Autodesk Fusion 360 part; units mm, degrees
(part 3 of 5)
fillet "Fillet8" radius 2.5 2 edges at (-19.3, 26.725, 15) (19.3, 26.725, 15)
fillet "Fillet9" radius 2.5 4 edges at (20.0322, 25.9928, 10) (19.3, 24, 10) (-19.3, 24, 10) (-20.0322, 25.9928, 10)
fillet "Fillet10" radius 15 2 edges at (29.0855, 18.4895, 0) (-29.0855, 18.4895, 0)
sketch "Sketch20" plane through (0, 26.725, 0) normal (0, 1, 0) x (-1, 0, 0)
  line L0 (-21.8, 12.5) -> (-21.8, 20)
  line L1 (-21.8, 20) -> (-28.05, 20)
  line L2 (-28.05, 20) -> (-28.05, -20)
  line L3 (-28.05, -20) -> (28.05, -20)
  line L4 (28.05, -20) -> (28.05, 20)
  line L5 (28.05, 20) -> (21.8, 20)
  line L6 (21.8, 20) -> (21.8, 12.5)
  spline S0 degree 3 poles (17.4699, 10) (17.7885, 10) (18.1326, 10.0486) (18.7976, 10.2365) (19.1187, 10.3749) (19.8306, 10.7581) (20.2629, 11.0723) (21.0731, 11.7716) (21.4536, 12.1536) (21.8, 12.5) knots 1.263831 1.263831 1.263831 1.263831 1.35941 1.35941 1.454989 1.454989 1.601942 1.601942 1.748896 1.748896 1.748896 1.748896
  line L7 (17.4699, 10) -> (-17.4699, 10)
  spline S1 degree 3 poles (-21.8, 12.5) (-21.4536, 12.1536) (-21.0731, 11.7716) (-20.2629, 11.0723) (-19.8306, 10.7581) (-19.1187, 10.3749) (-18.7976, 10.2365) (-18.1326, 10.0486) (-17.7885, 10) (-17.4699, 10) knots 0 0 0 0 0.146954 0.146954 0.293907 0.293907 0.389486 0.389486 0.485065 0.485065 0.485065 0.485065
  line L8 (20, -20) -> (-20, -20)
  line L9 (-20, -20) -> (-20, -15)
  line L10 (-20, -15) -> (20, -15)
  line L11 (20, -15) -> (20, -20)
  dimension "d224" = 5
  dimension "d225" = 40
  dimension "d226" = 20
  constraint horizontal L8
  constraint vertical L9
  constraint horizontal L10
  constraint vertical L11
  constraint coincident L3 L8.start
  measures "d224" distance of L8 L10
  measures "d225" distance of L9 L11
  measures "d226" distance of origin L9
extrude "Extrude19" add sketch "Sketch20" along normal blind 7.05 contours L3 L8 L9 L10 L11
fillet "Fillet11" radius 2.5 2 edges at (-20, 26.725, -17.5) (-20, 33.775, -17.5)
fillet "Fillet11" radius 2.5 2 edges at (20, 33.775, -17.5) (20, 26.725, -17.5)
fillet "Fillet12" radius 2.5 1 edges at (0, 26.725, -15)
sketch "Sketch21" plane through (0, 26.725, 0) normal (0, 1, 0) x (-1, 0, 0)
  line L0 (22.5, -12.5) -> (22.5, -20)
  line L1 (22.5, -20) -> (28.05, -20)
  line L2 (28.05, -20) -> (28.05, 20)
  line L3 (28.05, 20) -> (21.8, 20)
  line L4 (21.8, 20) -> (21.8, 12.5)
  spline S0 degree 3 poles (17.4699, 10) (17.7885, 10) (18.1326, 10.0486) (18.7976, 10.2365) (19.1187, 10.3749) (19.8306, 10.7581) (20.2629, 11.0723) (21.0731, 11.7716) (21.4536, 12.1536) (21.8, 12.5) knots 1.263831 1.263831 1.263831 1.263831 1.35941 1.35941 1.454989 1.454989 1.601942 1.601942 1.748896 1.748896 1.748896 1.748896
  line L5 (17.4699, 10) -> (-17.4699, 10)
  spline S1 degree 3 poles (-21.8, 12.5) (-21.4536, 12.1536) (-21.0731, 11.7716) (-20.2629, 11.0723) (-19.8306, 10.7581) (-19.1187, 10.3749) (-18.7976, 10.2365) (-18.1326, 10.0486) (-17.7885, 10) (-17.4699, 10) knots 0 0 0 0 0.146954 0.146954 0.293907 0.293907 0.389486 0.389486 0.485065 0.485065 0.485065 0.485065
  line L6 (-21.8, 12.5) -> (-21.8, 20)
  line L7 (-21.8, 20) -> (-28.05, 20)
  line L8 (-28.05, 20) -> (-28.05, -20)
  line L9 (-28.05, -20) -> (-22.5, -20)
  line L10 (-22.5, -20) -> (-22.5, -12.5)
  line L11 (-22.5, -12.5) -> (22.5, -12.5)
  line L12 (16.8, -6.4222) -> (16.8, 3.9222)
  line L13 (-16.8, -6.4222) -> (-16.8, 3.9222)
  line L14 (12.6427, 7.5) -> (-12.6427, 7.5)
  line L15 (12.6427, -10) -> (-12.6427, -10)
  line L16 (-19.3, 12.5) -> (-19.3, 20)
  line L17 (19.3, 20) -> (19.3, 12.5)
  line L18 (12.8627, 6.551) -> (1.3198, 0.8965)
  line L19 (-1.3198, 0.8965) -> (-12.8627, 6.551)
  line L20 (-15.3731, 4.8265) -> (-4.4158, -0.3457)
  line L21 (-4.4158, -2.1543) -> (-15.3731, -7.3265)
  line L22 (-12.8627, -9.051) -> (-1.3198, -3.3965)
  line L23 (1.3198, -3.3965) -> (12.8627, -9.051)
  line L24 (15.3731, -7.3265) -> (4.4158, -2.1543)
  line L25 (4.4158, -0.3457) -> (15.3731, 4.8265)
  arc A0 (4.4158, -0.3457) -> (4.4158, -2.1543) centre (4.8427, -1.25) ccw
  arc A1 (-4.4158, -2.1543) -> (-4.4158, -0.3457) centre (-4.8427, -1.25) ccw
  arc A2 (-1.3198, 0.8965) -> (1.3198, 0.8965) centre (0, 3.5906) ccw
  arc A3 (1.3198, -3.3965) -> (-1.3198, -3.3965) centre (0, -6.0906) ccw
  arc A4 (12.6427, -10) -> (12.8627, -9.051) centre (12.6427, -9.5) ccw
  arc A5 (-12.8627, -9.051) -> (-12.6427, -10) centre (-12.6427, -9.5) ccw
  arc A6 (-12.6427, 7.5) -> (-12.8627, 6.551) centre (-12.6427, 7) ccw
  arc A7 (12.8627, 6.551) -> (12.6427, 7.5) centre (12.6427, 7) ccw
  arc A8 (15.3731, -7.3265) -> (16.8, -6.4222) centre (15.8, -6.4222) ccw
  arc A9 (16.8, 3.9222) -> (15.3731, 4.8265) centre (15.8, 3.9222) ccw
  arc A10 (-15.3731, 4.8265) -> (-16.8, 3.9222) centre (-15.8, 3.9222) ccw
  arc A11 (-16.8, -6.4222) -> (-15.3731, -7.3265) centre (-15.8, -6.4222) ccw
  point P0 (-16.8, -8)
  point P1 (-16.8, 5.5)
  point P2 (14.8, 7.5)
  point P3 (-14.8, 7.5)
  point P4 (-14.8, -10)
  point P5 (0, -2.75)
  point P6 (0, 0.25)
  point P7 (-2.5, -1.25)
  point P8 (2.5, -1.25)
  dimension "d235" = 2.5
  dimension "d236" = 2.5
  dimension "d237" = 2.5
  dimension "d238" = 2.5
  dimension "d239" = 3
  dimension "d240" = 5
  dimension "d241" = 2.5
  dimension "d243" = 7.25
  dimension "d244" = 1.5
  dimension "d245" = 2
  dimension "d246" = 2
  dimension "d247" = 2
  dimension "d248" = 2
  dimension "d249" = 1
  dimension "d250" = 3
  dimension "d251" = 0.5
  dimension "d252" = 1
  constraint perpendicular L11 L12
  constraint vertical L13
  constraint horizontal L14
  constraint horizontal L15
  constraint vertical P5 P6
  constraint vertical origin P5
  constraint horizontal P7 P8
  constraint vertical P3 P4
  constraint tangent L24 A0
  constraint tangent L25 A0
  constraint tangent L21 A1
  constraint tangent L20 A1
  constraint equal A0 A1
  constraint tangent L18 A2
  constraint tangent L19 A2
  constraint tangent L23 A3
  constraint tangent L22 A3
  constraint equal A2 A3
  constraint tangent L23 A4
  constraint tangent L15 A4
  constraint coincident P4 L15
  constraint coincident P4 L22
  constraint tangent L15 A5
  constraint tangent L22 A5
  constraint equal A4 A5
  constraint coincident P3 L19
  constraint coincident P3 L14
  constraint tangent L19 A6
  constraint tangent L14 A6
  constraint equal A4 A6
  constraint coincident P2 L14
  constraint coincident P2 L18
  constraint tangent L14 A7
  constraint tangent L18 A7
  constraint equal A4 A7
  constraint tangent L24 A8
  constraint tangent L12 A8
  constraint tangent L12 A9
  constraint tangent L25 A9
  constraint equal A8 A9
  constraint coincident P1 L20
  constraint coincident P1 L13
  constraint tangent L20 A10
  constraint tangent L13 A10
  constraint equal A8 A10
  constraint coincident P0 L13
  constraint coincident P0 L21
  constraint tangent L13 A11
  constraint tangent L21 A11
  constraint equal A8 A11
  measures "d235" distance of L11 L15
  measures "d236" distance of L5 L14
  measures "d237" distance of L13 L16
  measures "d238" distance of L12 L17
  measures "d239" distance of P5 P6
  measures "d240" distance of P7 P8
  measures "d241" horizontal distance of origin P7
  measures "d243" distance of L14 P6
  measures "d244" vertical distance of P6 P7
  measures "d245" distance of L12 P2
  measures "d246" horizontal distance of P1 P3
  measures "d247" vertical distance of P0 P4
  measures "d248" vertical distance of P1 P3
  measures "d249" radius of A0
  measures "d250" radius of A2
  measures "d251" radius of A4
  measures "d252" radius of A8
extrude "Extrude20" cut sketch "Sketch21" against normal blind 0.45 contours L12 L24 L25 A0 A8 A9 | L13 L20 L21 A1 A10 A11 | L14 L18 L19 A2 A6 A7 | L15 L22 L23 A3 A4 A5
equation "d4 = ( 52.55 / 2 ) * 1 mm"
equation "d8 = ( 57.1 / 2 ) * 1 mm"
equation "d20 = 3.75 mm + 2.5 mm - 0.45 mm"
equation "d88 = ( ( 20.1 - 14 ) / 2 ) * 1 mm"
equation "d102 = ( 45 / 2 ) * 1 mm"
equation "d243 = ( ( 17.5 - 3 ) / 2 ) * 1 mm"

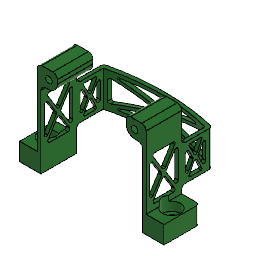
design "LGR RM Back Holder (Goalie)"
Autodesk Fusion 360 part; units mm, degrees
sketch "Sketch1" plane through (0, 0, 0) normal (0, 0, 1) x (1, 0, 0)
  line L0 (-30.55, 35) -> (-28.55, 35)
  line L1 (-28.55, 35) -> (-28.55, 0)
  line L2 (-28.55, 0) -> (-30.55, 0)
  line L3 (-30.55, 0) -> (-30.55, 35)
  line L4 (28.55, 35) -> (30.55, 35)
  line L5 (30.55, 35) -> (30.55, 0)
  line L6 (30.55, 0) -> (28.55, 0)
  line L7 (28.55, 0) -> (28.55, 35)
  dimension "d1" = 35
  dimension "d2" = 35
  dimension "d3" = 2
  dimension "d4" = 2
  dimension "d5" = 57.1
  dimension "d6" = 28.55
  constraint horizontal L0
  constraint vertical L1
  constraint horizontal L2
  constraint vertical L3
  constraint horizontal L4
  constraint vertical L5
  constraint horizontal L6
  constraint vertical L7
  constraint horizontal L0.start L4.start
  constraint horizontal origin L1.end
  measures "d1" distance of L0 L2
  measures "d2" distance of L4 L6
  measures "d3" distance of L1 L3
  measures "d4" distance of L5 L7
  measures "d5" distance of L1 L7
  measures "d6" distance of origin L7
extrude "Extrude1" add sketch "Sketch1" along normal blind 20 makes body 1 at (-28.55, 23.3333, 13.3333) makes body 2 at (30.55, 23.3333, 13.3333)
sketch "Sketch3" plane through (0, 0, 20) normal (0, 0, 1) x (-1, 0, 0)
  line L0 (-28.55, 0) -> (-30.55, 0)
  line L1 (-30.55, 0) -> (-30.55, -35)
  line L2 (-30.55, -35) -> (-28.55, -35)
  line L3 (-28.55, -35) -> (-28.55, 0)
  arc A0 (-28.55, -35) -> (28.55, -35) centre (0, 73.299) ccw
  arc A1 (-30.55, -37) -> (30.55, -37) centre (0, 87.272) ccw
  line L4 (30.55, -37) -> (30.55, -35)
  line L5 (-30.55, -37) -> (-30.55, -35)
  line L6 (-28.55, -35) -> (-30.55, -35)
  line L7 (28.55, -35) -> (30.55, -35)
  point P0 (-28.55, -35)
  point P1 (28.55, -35)
  point P2 (0, -38.7)
  point P3 (0, -40.7)
  point P4 (30.55, -37)
  point P5 (-30.55, -37)
  point P6 (30.55, -35)
  point P7 (28.55, -35)
  dimension "d9" = 3.7
  dimension "d10" = 2
  dimension "d11" = 2
  dimension "d12" = 2
  constraint coincident P0 L2.end
  constraint coincident P2 A0
  constraint coincident P7 P1
  constraint vertical origin P2
  constraint vertical P2 P3
  constraint vertical L1.end P5
  constraint vertical P4 P6
  constraint coincident P3 A1
  constraint coincident P5 A1.start
  constraint coincident P4 A1.end
  constraint coincident P6 L4.end
  constraint coincident L1.end L2.start
  measures "d9" vertical distance of P0 P2
  measures "d10" distance of P2 P3
  measures "d11" distance of P4 P6
  measures "d12" distance of L1.end P5
extrude "Extrude2" add sketch "Sketch3" against normal blind 20 contours L2 A0 A1 L4 L5 L6 L7 bodies 1 2
sketch "Sketch4" plane through (30.55, 0, 0) normal (1, 0, 0) x (0, 1, 0)
  line L0 (0, 0) -> (37, 0)
  line L1 (37, 0) -> (37, 20)
  line L2 (37, 20) -> (0, 20)
  line L3 (0, 20) -> (0, 0)
  line L4 (0, 0) -> (20, 0)
  line L5 (20, 0) -> (20, -4)
  line L6 (20, -4) -> (0, -4)
  line L7 (0, -4) -> (0, 0)
  dimension "d15" = 4
  dimension "d16" = 20
  constraint horizontal L4
  constraint vertical L5
  constraint horizontal L6
  constraint vertical L7
  constraint coincident L0.start L3.end
  measures "d15" distance of L4 L6
  measures "d16" distance of L5 L7
extrude "Extrude3" add sketch "Sketch4" against normal blind 2 contours L0 L4 L5 L6 L7 bodies 1
sketch "Sketch5" plane through (-30.55, 0, 0) normal (-1, 0, 0) x (0, -1, 0)
  line L0 (-37, 0) -> (0, 0)
  line L1 (0, 0) -> (0, 20)
  line L2 (0, 20) -> (-37, 20)
  line L3 (-37, 20) -> (-37, 0)
  line L4 (0, 0) -> (-20, 0)
  line L5 (-20, 0) -> (-20, -4)
  line L6 (-20, -4) -> (0, -4)
  line L7 (0, -4) -> (0, 0)
  dimension "d19" = 4
  dimension "d20" = 20
  constraint horizontal L4
  constraint vertical L5
  constraint horizontal L6
  constraint vertical L7
  constraint coincident L0.end L1.start
  measures "d19" distance of L4 L6
  measures "d20" distance of L5 L7
extrude "Extrude4" add sketch "Sketch5" against normal blind 2 contours L0 L4 L5 L6 L7 bodies 1
sketch "Sketch6" plane through (0, 0, 0) normal (0, -1, 0) x (1, 0, 0)
  line L0 (30.55, -4) -> (30.55, 20)
  line L1 (30.55, 20) -> (28.55, 20)
  line L2 (28.55, 20) -> (28.55, -4)
  line L3 (28.55, -4) -> (30.55, -4)
  line L4 (28.55, -4) -> (40.55, -4)
  line L5 (40.55, -4) -> (40.55, -14)
  line L6 (40.55, -14) -> (28.55, -14)
  line L7 (28.55, -14) -> (28.55, -4)
  line L8 (-28.55, -4) -> (-40.55, -4)
  line L9 (-40.55, -4) -> (-40.55, -14)
  line L10 (-40.55, -14) -> (-28.55, -14)
  line L11 (-28.55, -14) -> (-28.55, -4)
  dimension "d23" = 57.1
  dimension "d24" = 12
  dimension "d25" = 10
  dimension "d26" = 12
  constraint horizontal L4
  constraint vertical L5
  constraint horizontal L6
  constraint vertical L7
  constraint coincident L2.end L3.start
  constraint horizontal L8
  constraint vertical L9
  constraint horizontal L10
  constraint vertical L11
  constraint horizontal L6.end L10.end
  constraint horizontal L2.end L8.start
  measures "d23" distance of L2.end L8.start
  measures "d24" distance of L5 L7
  measures "d25" distance of L4 L6
  measures "d26" distance of L9 L11
extrude "Extrude5" add sketch "Sketch6" against normal blind 20 contours L3 L4 L5 L6 L7 | L8 L9 L10 L11 bodies 1
sketch "Sketch7" plane through (0, 0, -4) normal (0, 0, 1) x (-1, 0, 0)
  line L0 (-30.55, -20) -> (-30.55, 0)
  line L1 (-30.55, 0) -> (-40.55, 0)
  line L2 (-40.55, 0) -> (-40.55, -20)
  line L3 (-40.55, -20) -> (-30.55, -20)
  line L4 (40.55, 0) -> (40.55, -20)
  point P0 (-34.75, -10)
  point P1 (34.75, -10)
  dimension "d29" = 5.8
  dimension "d30" = 5.8
  dimension "d31" = 10
  constraint horizontal P0 P1
  measures "d29" distance of L2 P0
  measures "d30" distance of P1 L4
  measures "d31" distance of L1 P0
hole "Hole1" at (34.75, 10, -4) at (-34.75, 10, -4) direction (0, 0, -1) diameter 5.3 depth 20 tip angle 180 counterbore diameter 10 counterbore depth 5 bodies 1
fillet "Fillet1" radius 2 2 edges at (40.55, 20, -9) (-40.55, 20, -9) on bodies 1
fillet "Fillet2" radius 2 4 edges at (30.55, 37, 10) (-30.55, 37, 10) (29.55, 20, 0) (-29.55, 20, 0) on bodies 1
sketch "Sketch8" plane through (0, 0, 0) normal (0, -1, 0) x (1, 0, 0)
  line L0 (30.55, -4) -> (30.55, 20)
  line L1 (30.55, 20) -> (28.55, 20)
  line L2 (28.55, 20) -> (28.55, -14)
  line L3 (28.55, -14) -> (40.55, -14)
  line L4 (40.55, -14) -> (40.55, -4)
  line L5 (40.55, -4) -> (30.55, -4)
  line L6 (30.55, 20) -> (28.55, 20)
  line L7 (30.55, 36.5) -> (30.55, 20)
  line L8 (-30.55, 20) -> (-28.55, 20)
  line L9 (-30.55, 36.5) -> (-30.55, 20)
  line L10 (28.55, 20) -> (-28.55, 20)
  line L11 (-19.3, 36.5) -> (-19.3, 34.25)
  line L12 (-24.3, 29.25) -> (-26.05, 29.25)
  line L13 (19.3, 36.5) -> (19.3, 34.25)
  line L14 (24.3, 29.25) -> (26.05, 29.25)
  line L15 (-28.55, 26.75) -> (-28.55, 20)
  line L16 (28.55, 26.75) -> (28.55, 20)
  line L17 (-28.05, 39) -> (-21.8, 39)
  line L18 (21.8, 39) -> (28.05, 39)
  arc A0 (30.55, 36.5) -> (28.05, 39) centre (28.05, 36.5) ccw
  arc A1 (-28.05, 39) -> (-30.55, 36.5) centre (-28.05, 36.5) ccw
  arc A2 (21.8, 39) -> (19.3, 36.5) centre (21.8, 36.5) ccw
  arc A3 (28.55, 26.75) -> (26.05, 29.25) centre (26.05, 26.75) ccw
  arc A4 (-26.05, 29.25) -> (-28.55, 26.75) centre (-26.05, 26.75) ccw
  arc A5 (-19.3, 36.5) -> (-21.8, 39) centre (-21.8, 36.5) ccw
  arc A6 (19.3, 34.25) -> (24.3, 29.25) centre (24.3, 34.25) ccw
  arc A7 (-24.3, 29.25) -> (-19.3, 34.25) centre (-24.3, 34.25) ccw
  point P0 (-30.55, 39)
  point P1 (-19.3, 39)
  point P2 (-19.3, 29.25)
  point P3 (-28.55, 29.25)
  point P4 (19.3, 39)
  point P5 (19.3, 29.25)
  point P6 (28.55, 29.25)
  dimension "d41" = 61.1
  dimension "d51" = 9.75
  dimension "d52" = 9.75
  dimension "d53" = 9.25
  dimension "d54" = 9.25
  dimension "d55" = 11.25
  dimension "d56" = 9.25
  dimension "d57" = 2.5
  dimension "d58" = 2.5
  dimension "d59" = 5
  constraint horizontal L6
  constraint vertical L7
  constraint coincident L0.end L1.start
  constraint horizontal L8
  constraint vertical L9
  constraint horizontal L0.end L8.start
  constraint vertical L11
  constraint horizontal L12
  constraint vertical L13
  constraint horizontal L14
  constraint perpendicular L10 L15
  constraint coincident L1.end L2.start
  constraint perpendicular L6 L16
  constraint perpendicular L11 L17
  constraint horizontal P2 P5
  constraint tangent L18 A0
  constraint tangent L7 A0
  constraint coincident P0 L17
  constraint coincident P0 L9
  constraint tangent L17 A1
  constraint tangent L9 A1
  constraint equal A0 A1
  constraint coincident P4 L13
  constraint coincident P4 L18
  constraint tangent L13 A2
  constraint tangent L18 A2
  constraint coincident P6 L14
  constraint coincident P6 L16
  constraint tangent L14 A3
  constraint tangent L16 A3
  constraint equal A2 A3
  constraint coincident P3 L12
  constraint coincident P3 L15
  constraint tangent L12 A4
  constraint tangent L15 A4
  constraint equal A2 A4
  constraint coincident P1 L11
  constraint coincident P1 L17
  constraint tangent L11 A5
  constraint tangent L17 A5
  constraint equal A2 A5
  constraint coincident P5 L14
  constraint coincident P5 L13
  constraint tangent L14 A6
  constraint tangent L13 A6
  constraint coincident P2 L12
  constraint coincident P2 L11
  constraint tangent L12 A7
  constraint tangent L11 A7
  constraint equal A6 A7
  measures "d41" distance of L0.end L8.start
  measures "d51" distance of P1 P2
  measures "d52" distance of P4 P5
  measures "d53" distance of P2 P3
  measures "d54" distance of P5 P6
  measures "d55" distance of P0 P1
  measures "d56" distance of P6 L1.end
  measures "d57" radius of A0
  measures "d58" radius of A2
  measures "d59" radius of A6
extrude "Extrude6" add sketch "Sketch8" against normal blind 20 contours L1 L6 L7 L13 L14 L16 L18 A0 A2 A3 A6 | L8 L9 L11 L12 L15 L17 A1 A4 A5 A7 bodies 1
sketch "Sketch9" plane through (0, 20, 0) normal (0, 1, 0) x (-1, 0, 0)
  arc A0 (-19.3, 36.5) -> (-21.8, 39) centre (-21.8, 36.5) ccw
  line L0 (-21.8, 39) -> (-28.05, 39)
  arc A1 (-28.05, 39) -> (-30.55, 36.5) centre (-28.05, 36.5) ccw
  line L1 (-30.55, 36.5) -> (-30.55, 20)
  line L2 (-30.55, 20) -> (-28.55, 20)
  line L3 (-28.55, 20) -> (-28.55, 26.75)
  arc A2 (-26.05, 29.25) -> (-28.55, 26.75) centre (-26.05, 26.75) ccw
  line L4 (-26.05, 29.25) -> (-24.3, 29.25)
  arc A3 (-24.3, 29.25) -> (-19.3, 34.25) centre (-24.3, 34.25) ccw
  line L5 (-19.3, 34.25) -> (-19.3, 36.5)
  line L6 (30.55, 20) -> (30.55, 36.5)
  point P0 (-24.05, 34.05)
  point P1 (24.05, 34.05)
  dimension "d62" = 6.5
  dimension "d63" = 6.5
  dimension "d64" = 4.95
  constraint horizontal P0 P1
  measures "d62" distance of L1 P0
  measures "d63" distance of P1 L6
  measures "d64" distance of L0 P0
hole "Hole3" at (24.05, 20, 34.05) at (-24.05, 20, 34.05) direction (0, -1, 0) diameter 6.5 depth 12.5 tip angle 180 bodies 1
sketch "Sketch10" plane through (0, 7.5, 0) normal (0, 1, 0) x (-1, 0, 0)
  circle A0 centre (-24.05, 34.05) radius 3.25
  line L0 (-30.55, 36.5) -> (-30.55, 20)
  line L1 (30.55, 20) -> (30.55, 36.5)
  line L2 (-21.8, 39) -> (-28.05, 39)
  point P0 (-24.05, 34.05)
  point P1 (24.05, 34.05)
  dimension "d73" = 6.5
  dimension "d74" = 6.5
  dimension "d75" = 4.95
  constraint horizontal P0 P1
  measures "d73" distance of P0 L0
  measures "d74" distance of P1 L1
  measures "d75" distance of P0 L2
hole "Hole4" at (24.05, 7.5, 34.05) at (-24.05, 7.5, 34.05) direction (0, -1, 0) diameter 3.6 end through all counterbore diameter 6.5 counterbore depth 3 bodies 1
sketch "Sketch11" plane through (30.55, 0, 0) normal (1, 0, 0) x (0, 1, 0)
  line L0 (35.4221, 0) -> (35.4221, 20)
  line L1 (35.4221, 20) -> (20, 20)
  line L2 (20, 20) -> (20, 36.5)
  line L3 (20, 36.5) -> (0, 36.5)
  line L4 (0, 36.5) -> (0, -4)
  line L5 (0, -4) -> (7.2871, -4)
  line L6 (7.2871, -4) -> (12.7129, -4)
  line L7 (12.7129, -4) -> (20, -4)
  line L8 (20, -4) -> (20, -2)
  arc A0 (22, 0) -> (20, -2) centre (22, -2) ccw
  line L9 (22, 0) -> (35.4221, 0)
  arc A1 (8.659, 10.728) -> (8.6579, 11.8018) centre (7.8148, 11.264) ccw
  line L10 (8.659, 10.728) -> (3.8443, 3.1449)
  line L11 (3.8432, 19.3505) -> (8.6579, 11.8018)
  line L12 (0.0001, 38.0402) -> (0.0001, -4.0098)
  arc A2 (3.8432, 19.3505) -> (2.0001, 18.8128) centre (3.0001, 18.8128) ccw
  arc A3 (2.0001, 3.6809) -> (3.8443, 3.1449) centre (3.0001, 3.6809) ccw
  arc A4 (18.0001, 18.8128) -> (16.157, 19.3505) centre (17.0001, 18.8128) ccw
  line L13 (16.088, 21.9584) -> (10.853, 13.6232)
  line L14 (9.1559, 13.6286) -> (3.9952, 21.9638)
  line L15 (3.99, 0.515) -> (9.1549, 8.8941)
  line L16 (15.2412, 23.4902) -> (4.8454, 23.4902)
  line L17 (2.0001, 18.8128) -> (2.0001, 3.6809)
  arc A5 (10.8541, 8.8995) -> (9.1549, 8.8941) centre (10.0062, 8.3693) ccw
  line L18 (20.0001, 40.5402) -> (0.0001, 40.5402)
  arc A6 (3.99, 0.515) -> (4.8412, -1.0098) centre (4.8412, -0.0098) ccw
  line L19 (20.0001, 38.0402) -> (0.0001, 38.0402)
  arc A7 (4.8454, 23.4902) -> (3.9952, 21.9638) centre (4.8454, 22.4902) ccw
  line L20 (15.2454, -1.0098) -> (4.8412, -1.0098)
  line L21 (18.0001, 18.8128) -> (18.0001, 3.6809)
  arc A8 (16.088, 21.9584) -> (15.2412, 23.4902) centre (15.2412, 22.4902) ccw
  line L22 (16.1559, 3.1449) -> (11.3412, 10.728)
  arc A9 (9.1559, 13.6286) -> (10.853, 13.6232) centre (10.0062, 14.1551) ccw
  line L23 (10.8541, 8.8995) -> (16.0933, 0.5204)
  line L24 (11.3423, 11.8018) -> (16.157, 19.3505)
  arc A10 (11.3423, 11.8018) -> (11.3412, 10.728) centre (12.1854, 11.264) ccw
  line L25 (12.713, -4.0098) -> (20.0001, -4.0098)
  arc A11 (16.1559, 3.1449) -> (18.0001, 3.6809) centre (17.0001, 3.6809) ccw
  arc A12 (15.2454, -1.0098) -> (16.0933, 0.5204) centre (15.2454, -0.0098) ccw
  line L26 (0.0001, -4.0098) -> (7.2872, -4.0098)
  line L27 (20.0001, -4.0098) -> (20.0001, 38.0402)
  point P0 (9.0001, 11.2652)
  point P1 (11.0001, 11.2652)
  point P2 (18.0001, 0.2402)
  point P3 (2.0001, 22.2402)
  point P4 (10.0001, 10.2652)
  point P5 (10.0501, 11.2402)
  point P6 (17.0501, 23.4902)
  point P7 (2.0001, 0.2402)
  point P8 (3.0501, -1.0098)
  point P9 (17.0501, -1.0098)
  point P10 (3.0501, 23.4902)
  point P11 (10.0001, 12.2652)
  point P12 (0.0001, 12.2652)
  point P13 (18.0001, 22.2402)
  dimension "d80" = 3
  dimension "d81" = 17.05
  dimension "d82" = 2
  dimension "d83" = 2
  dimension "d86" = 22
  dimension "d87" = 22
  dimension "d88" = 14
  dimension "d89" = 14
  dimension "d90" = 4.25
  dimension "d91" = 3.05
  dimension "d92" = 1
  constraint perpendicular L16 L27
  constraint perpendicular L16 L17
  constraint coincident P6 L13
  constraint coincident P6 L16
  constraint tangent L13 A8
  constraint tangent L16 A8
  constraint coincident P10 L16
  constraint coincident P10 L14
  constraint tangent L16 A7
  constraint tangent L14 A7
  constraint equal A7 A8
  constraint tangent L14 A9
  constraint tangent L13 A9
  constraint equal A8 A9
  constraint tangent A1 L11
  constraint tangent A1 L10
  constraint equal A1 A8
  constraint coincident P7 L10
  constraint coincident P7 L17
  constraint tangent L10 A3
  constraint tangent A3 L17
  constraint equal A3 A8
  constraint coincident P3 L17
  constraint coincident P3 L11
  constraint tangent A2 L17
  constraint tangent L11 A2
  constraint equal A2 A8
  constraint coincident P8 L15
  constraint coincident P8 L20
  constraint tangent L15 A6
  constraint tangent A6 L20
  constraint equal A6 A8
  constraint coincident P9 L20
  constraint coincident P9 L23
  constraint tangent L20 A12
  constraint tangent L23 A12
  constraint equal A8 A12
  constraint coincident P2 L22
  constraint coincident P2 L21
  constraint tangent L22 A11
  constraint tangent L21 A11
  constraint equal A8 A11
  constraint coincident P13 L24
  constraint coincident P13 L21
  constraint tangent A4 L24
  constraint tangent A4 L21
  constraint equal A4 A8
  constraint tangent L22 A10
  constraint tangent L24 A10
  constraint equal A8 A10
  constraint tangent L15 A5
  constraint tangent A5 L23
  constraint equal A5 A8
  measures "d80" distance of L20 L25
  measures "d81" distance of L16 L18
  measures "d82" distance of L21 L27
  measures "d83" distance of L12 L17
  measures "d86" distance of P2 P13
  measures "d87" distance of P3 P7
  measures "d88" distance of P8 P9
  measures "d89" distance of P6 P10
  measures "d90" distance of P2 L25
  measures "d91" distance of P8 L12
  measures "d92" radius of A8
extrude "Extrude7" cut sketch "Sketch11" against normal blind 65 contours A1 L10 L11 A2 A3 L17 | A4 L21 L22 L24 A10 A11 | L13 L14 L16 A7 A8 A9 | L15 A5 A6 L20 L23 A12 bodies 1
sketch "Sketch12" plane through (30.55, 0, 0) normal (1, 0, 0) x (0, 1, 0)
  line L0 (16.1559, 3.1449) -> (11.3412, 10.728)
  arc A0 (11.3423, 11.8018) -> (11.3412, 10.728) centre (12.1854, 11.264) ccw
  line L1 (11.3423, 11.8018) -> (16.157, 19.3505)
  arc A1 (18.0001, 18.8128) -> (16.157, 19.3505) centre (17.0001, 18.8128) ccw
  line L2 (18.0001, 18.8128) -> (18.0001, 3.6809)
  arc A2 (16.1559, 3.1449) -> (18.0001, 3.6809) centre (17.0001, 3.6809) ccw
  line L3 (15.2454, -1.0098) -> (4.8412, -1.0098)
  arc A3 (3.99, 0.515) -> (4.8412, -1.0098) centre (4.8412, -0.0098) ccw
  line L4 (3.99, 0.515) -> (9.1549, 8.8941)
  arc A4 (10.8541, 8.8995) -> (9.1549, 8.8941) centre (10.0062, 8.3693) ccw
  line L5 (10.8541, 8.8995) -> (16.0933, 0.5204)
  arc A5 (15.2454, -1.0098) -> (16.0933, 0.5204) centre (15.2454, -0.0098) ccw
  line L6 (4.8454, 23.4902) -> (15.2412, 23.4902)
  arc A6 (16.088, 21.9584) -> (15.2412, 23.4902) centre (15.2412, 22.4902) ccw
  line L7 (16.088, 21.9584) -> (10.853, 13.6232)
  arc A7 (9.1559, 13.6286) -> (10.853, 13.6232) centre (10.0062, 14.1551) ccw
  line L8 (9.1559, 13.6286) -> (3.9952, 21.9638)
  arc A8 (4.8454, 23.4902) -> (3.9952, 21.9638) centre (4.8454, 22.4902) ccw
  line L9 (2.0001, 3.6809) -> (2.0001, 18.8128)
  arc A9 (3.8432, 19.3505) -> (2.0001, 18.8128) centre (3.0001, 18.8128) ccw
  line L10 (3.8432, 19.3505) -> (8.6579, 11.8018)
  arc A10 (8.659, 10.728) -> (8.6579, 11.8018) centre (7.8148, 11.264) ccw
  line L11 (8.659, 10.728) -> (3.8443, 3.1449)
  arc A11 (2.0001, 3.6809) -> (3.8443, 3.1449) centre (3.0001, 3.6809) ccw
  line L12 (35.4221, 0) -> (35.4221, 20)
  line L13 (35.4221, 20) -> (20, 20)
  line L14 (20, 20) -> (20, 36.5)
  line L15 (20, 36.5) -> (0, 36.5)
  line L16 (0, 36.5) -> (0, -4)
  line L17 (0, -4) -> (7.2871, -4)
  line L18 (7.2871, -4) -> (12.7129, -4)
  line L19 (12.7129, -4) -> (20, -4)
  line L20 (20, -4) -> (20, -2)
  arc A12 (22, 0) -> (20, -2) centre (22, -2) ccw
  line L21 (22, 0) -> (35.4221, 0)
  line L22 (24.5001, 18) -> (30.9221, 18)
  line L23 (33.4221, 14.5) -> (33.4221, 5.5)
  line L24 (30.9221, 2) -> (24.5001, 2)
  line L25 (22.0001, 5.5) -> (22.0001, 14.5)
  line L26 (24.0538, 17.2746) -> (26.8184, 11.7993)
  line L27 (28.6038, 11.7993) -> (31.3684, 17.2746)
  line L28 (31.5294, 14.9507) -> (29.1435, 10.2254)
  line L29 (29.1435, 9.7746) -> (31.5294, 5.0493)
  line L30 (31.3684, 2.7254) -> (28.6038, 8.2007)
  line L31 (26.8184, 8.2007) -> (24.0538, 2.7254)
  line L32 (23.8928, 5.0493) -> (26.2787, 9.7746)
  line L33 (26.2787, 10.2254) -> (23.8928, 14.9507)
  arc A13 (23.8928, 14.9507) -> (22.0001, 14.5) centre (23.0001, 14.5) ccw
  arc A14 (22.0001, 5.5) -> (23.8928, 5.0493) centre (23.0001, 5.5) ccw
  arc A15 (31.5294, 5.0493) -> (33.4221, 5.5) centre (32.4221, 5.5) ccw
  arc A16 (33.4221, 14.5) -> (31.5294, 14.9507) centre (32.4221, 14.5) ccw
  arc A17 (26.2787, 9.7746) -> (26.2787, 10.2254) centre (25.8324, 10) ccw
  arc A18 (29.1435, 10.2254) -> (29.1435, 9.7746) centre (29.5898, 10) ccw
  arc A19 (24.0538, 2.7254) -> (24.5001, 2) centre (24.5001, 2.5) ccw
  arc A20 (30.9221, 2) -> (31.3684, 2.7254) centre (30.9221, 2.5) ccw
  arc A21 (31.3684, 17.2746) -> (30.9221, 18) centre (30.9221, 17.5) ccw
  arc A22 (24.5001, 18) -> (24.0538, 17.2746) centre (24.5001, 17.5) ccw
  arc A23 (26.8184, 11.7993) -> (28.6038, 11.7993) centre (27.7111, 12.25) ccw
  arc A24 (28.6038, 8.2007) -> (26.8184, 8.2007) centre (27.7111, 7.75) ccw
  point P0 (24, 18)
  point P1 (22.0001, 16)
  point P2 (22.0001, 4)
  point P3 (24, 2)
  point P4 (66, 18)
  point P5 (33.4221, 16)
  point P6 (33.4221, 4)
  point P7 (66, 2)
  point P8 (45, 10)
  point P9 (45, 12)
  point P10 (43, 10)
  point P11 (45, 8)
  point P12 (47, 10)
  dimension "d95" = 1
  dimension "d96" = 0.5
  dimension "d97" = 0.5
  dimension "d98" = 1
  dimension "d130" = 4
  dimension "d131" = 2
  dimension "d132" = 2
  dimension "d133" = 2
  dimension "d134" = 6.5
  dimension "d135" = 4.5
  dimension "d136" = 5.5
  dimension "d137" = 5.5
  dimension "d138" = 7.75
  constraint horizontal L22
  constraint vertical L23
  constraint horizontal L24
  constraint vertical L25
  constraint coincident L22 P0
  constraint coincident L25 P1
  constraint coincident L25 P2
  constraint coincident L24 P3
  constraint coincident L22 P4
  constraint coincident L23 P5
  constraint coincident L23 P6
  constraint coincident L24 P7
  constraint parallel L27 L28
  constraint parallel L26 L29
  constraint parallel L29 L30
  constraint parallel L28 L31
  constraint parallel L31 L32
  constraint parallel L30 L33
  constraint tangent L33 A13
  constraint tangent L25 A13
  constraint tangent L32 A14
  constraint tangent L25 A14
  constraint equal A13 A14
  constraint tangent L29 A15
  constraint tangent L23 A15
  constraint equal A13 A15
  constraint tangent L28 A16
  constraint tangent L23 A16
  constraint equal A13 A16
  constraint tangent L33 A17
  constraint tangent L32 A17
  constraint tangent L29 A18
  constraint tangent L28 A18
  constraint equal A17 A18
  constraint tangent L31 A19
  constraint tangent L24 A19
  constraint tangent L24 A20
  constraint tangent L30 A20
  constraint equal A19 A20
  constraint tangent L27 A21
  constraint tangent L22 A21
  constraint equal A19 A21
  constraint tangent L26 A22
  constraint tangent L22 A22
  constraint equal A19 A22
  constraint tangent L26 A23
  constraint tangent L27 A23
  constraint tangent L31 A24
  constraint tangent L30 A24
  constraint equal A23 A24
  constraint vertical A19.centre A22.centre
  constraint vertical A20.centre A21.centre
  constraint horizontal A14.centre A15.centre
  constraint horizontal A13.centre A16.centre
  constraint vertical A23.centre A24.centre
  measures "d95" radius of A13
  measures "d96" radius of A17
  measures "d97" radius of A19
  measures "d98" radius of A23
  measures "d130" distance of L2 L25
  measures "d131" distance of L13 L22
  measures "d132" distance of L21 L24
  measures "d133" distance of L12 L23
  measures "d134" distance of L2 A22.centre
  measures "d135" distance of L12 A21.centre
  measures "d136" distance of L13 A13.centre
  measures "d137" distance of L21 A14.centre
  measures "d138" distance of L13 A23.centre
extrude "Extrude8" cut sketch "Sketch12" against normal blind 65 contours L22 L26 L27 A21 A22 A23 | L23 L28 L29 A15 A16 A18 | L24 L30 L31 A19 A20 A24 | L25 L32 L33 A13 A14 A17 bodies 1
sketch "Sketch15" plane through (0, 0, 0) normal (0, -1, 0) x (1, 0, 0)
  circle A0 centre (-24.05, 34.05) radius 1.8
  line L0 (-28.55, -14) -> (-28.55, 26.75)
  arc A1 (-26.05, 29.25) -> (-28.55, 26.75) centre (-26.05, 26.75) ccw
  line L1 (-26.05, 29.25) -> (-24.3, 29.25)
  arc A2 (-24.3, 29.25) -> (-19.3, 34.25) centre (-24.3, 34.25) ccw
  line L2 (-19.3, 34.25) -> (-19.3, 36.5)
  arc A3 (-19.3, 36.5) -> (-21.8, 39) centre (-21.8, 36.5) ccw
  line L3 (-21.8, 39) -> (-28.05, 39)
  arc A4 (-28.05, 39) -> (-30.55, 36.5) centre (-28.05, 36.5) ccw
  line L4 (-30.55, 36.5) -> (-30.55, -4)
  line L5 (-30.55, -4) -> (-40.55, -4)
  line L6 (-40.55, -4) -> (-40.55, -14)
  line L7 (-40.55, -14) -> (-28.55, -14)
  line L8 (-21.4029, 18) -> (21.4029, 18)
  line L9 (26.55, 15.2137) -> (26.55, 4.7863)
  line L10 (21.4029, 2) -> (-21.4029, 2)
  line L11 (-26.55, 4.7863) -> (-26.55, 15.2137)
  line L12 (28.55, 0) -> (-28.55, 0)
  line L13 (28.55, 20) -> (-28.55, 20)
  line L14 (28.55, -14) -> (28.55, 26.75)
  line L15 (-21.527, 2.9844) -> (-1.241, 8.182)
  line L16 (1.241, 8.182) -> (21.527, 2.9844)
  line L17 (25.3035, 3.8171) -> (3.8571, 9.2732)
  line L18 (3.8571, 10.7268) -> (25.3035, 16.1829)
  line L19 (21.527, 17.0156) -> (1.241, 11.818)
  line L20 (-1.241, 11.818) -> (-21.527, 17.0156)
  line L21 (-25.3035, 16.1829) -> (-3.8571, 10.7268)
  line L22 (-3.8571, 9.2732) -> (-25.3035, 3.8171)
  arc A5 (-25.3035, 16.1829) -> (-26.55, 15.2137) centre (-25.55, 15.2137) ccw
  arc A6 (-26.55, 4.7863) -> (-25.3035, 3.8171) centre (-25.55, 4.7863) ccw
  arc A7 (25.3035, 3.8171) -> (26.55, 4.7863) centre (25.55, 4.7863) ccw
  arc A8 (26.55, 15.2137) -> (25.3035, 16.1829) centre (25.55, 15.2137) ccw
  arc A9 (-3.8571, 9.2732) -> (-3.8571, 10.7268) centre (-4.042, 10) ccw
  arc A10 (3.8571, 10.7268) -> (3.8571, 9.2732) centre (4.042, 10) ccw
  arc A11 (-21.527, 2.9844) -> (-21.4029, 2) centre (-21.4029, 2.5) ccw
  arc A12 (21.4029, 2) -> (21.527, 2.9844) centre (21.4029, 2.5) ccw
  arc A13 (21.527, 17.0156) -> (21.4029, 18) centre (21.4029, 17.5) ccw
  arc A14 (-21.4029, 18) -> (-21.527, 17.0156) centre (-21.4029, 17.5) ccw
  arc A15 (-1.241, 11.818) -> (1.241, 11.818) centre (0, 16.6615) ccw
  arc A16 (1.241, 8.182) -> (-1.241, 8.182) centre (0, 3.3385) ccw
  point P0 (-26.55, 18)
  point P1 (26.55, 18)
  point P2 (26.55, 2)
  point P3 (-25.05, 18)
  point P4 (-25.05, 2)
  point P5 (25.05, 18)
  point P6 (25.05, 2)
  point P7 (0, 10)
  point P8 (-26.55, 16.5)
  point P9 (-26.55, 3.5)
  point P10 (26.55, 16.5)
  point P11 (26.55, 3.5)
  point P12 (0, 8.5)
  point P13 (-1, 10)
  point P14 (0, 11.5)
  point P15 (1, 10)
  dimension "d102" = 2
  dimension "d103" = 2
  dimension "d104" = 2
  dimension "d105" = 2
  dimension "d106" = 1.5
  dimension "d107" = 1.5
  dimension "d108" = 1.5
  dimension "d109" = 1.5
  dimension "d110" = 26.55
  dimension "d112" = 1
  dimension "d113" = 0.75
  dimension "d114" = 0.5
  dimension "d115" = 3
  dimension "d117" = 1.5
  dimension "d118" = 5
  constraint horizontal L8
  constraint vertical L9
  constraint horizontal L10
  constraint vertical L11
  constraint coincident L8 P3
  constraint coincident L10 P4
  constraint coincident L8 P5
  constraint coincident L10 P6
  constraint coincident L11 P8
  constraint coincident L11 P9
  constraint coincident L9 P10
  constraint coincident L9 P11
  constraint vertical P3 P4
  constraint horizontal P8 P10
  constraint horizontal P9 P11
  constraint vertical P5 P6
  constraint coincident P0 L11
  constraint tangent L21 A5
  constraint tangent L11 A5
  constraint tangent L22 A6
  constraint tangent L11 A6
  constraint equal A5 A6
  constraint coincident P2 L9
  constraint tangent L17 A7
  constraint tangent L9 A7
  constraint equal A5 A7
  constraint coincident P1 L9
  constraint tangent L9 A8
  constraint tangent L18 A8
  constraint equal A5 A8
  constraint tangent L22 A9
  constraint tangent L21 A9
  constraint tangent L17 A10
  constraint tangent L18 A10
  constraint equal A9 A10
  constraint tangent L15 A11
  constraint tangent L10 A11
  constraint coincident P2 L10
  constraint tangent L16 A12
  constraint tangent L10 A12
  constraint equal A11 A12
  constraint coincident P1 L8
  constraint tangent L19 A13
  constraint tangent L8 A13
  constraint equal A11 A13
  constraint coincident P0 L8
  constraint tangent L20 A14
  constraint tangent L8 A14
  constraint equal A11 A14
  constraint vertical P12 P14
  constraint horizontal A9.centre A10.centre
  constraint vertical P7 P12
  constraint horizontal P7 A10.centre
  constraint tangent L20 A15
  constraint tangent L19 A15
  constraint tangent L15 A16
  constraint tangent L16 A16
  constraint equal A15 A16
  measures "d102" distance of L0 L11
  measures "d103" distance of L10 L12
  measures "d104" distance of L8 L13
  measures "d105" distance of L9 L14
  measures "d106" distance of P0 P3
  measures "d107" distance of P0 P8
  measures "d108" distance of P1 P5
  measures "d109" distance of P2 P11
  measures "d110" horizontal distance of P0 P7
  measures "d112" radius of A5
  measures "d113" radius of A9
  measures "d114" radius of A11
  measures "d115" distance of P12 P14
  measures "d117" distance of P7 P12
  measures "d118" radius of A15
extrude "Extrude9" cut sketch "Sketch15" against normal blind 80 contours L8 L19 L20 A13 A14 A15 | L9 L17 L18 A7 A8 A10 | L10 L15 L16 A11 A12 A16 | L11 L21 L22 A5 A6 A9 bodies 1
sketch "Sketch16" plane through (0, 0, -4) normal (0, 0, 1) x (-1, 0, 0)
  arc A0 (-40.55, -18) -> (-38.55, -20) centre (-38.55, -18) ccw
  line L0 (-38.55, -20) -> (-30.55, -20)
  line L1 (-30.55, -20) -> (-30.55, -12.7129)
  arc A1 (-30.55, -7.2871) -> (-30.55, -12.7129) centre (-34.75, -10) ccw
  line L2 (-30.55, -7.2871) -> (-30.55, 0)
  line L3 (-30.55, 0) -> (-40.55, 0)
  line L4 (-40.55, 0) -> (-40.55, -18)
  circle A2 centre (-34.75, -10) radius 5
  circle A3 centre (34.75, -10) radius 5
  dimension "d121" = 10
  dimension "d122" = 10
  dimension "d123" = 69.5
  constraint concentric A1 A2
  constraint horizontal A1.centre A3.centre
  measures "d121" diameter of A2
  measures "d122" diameter of A3
  measures "d123" horizontal distance of A1.centre A3.centre
extrude "Extrude10" cut sketch "Sketch16" along normal blind 5 contours A1 A2 | A3 bodies 1
fillet "Fillet3" radius 2 2 edges at (29.55, 20, 20) (-29.55, 20, 20) on bodies 1
equation "d6 = ( 57.1 / 2 ) * 1 mm"
equation "d64 = 6.5 mm - 1.55 mm"
equation "d75 = 6.5 mm - 1.55 mm"
equation "d110 = ( 53.1 / 2 ) * 1 mm"

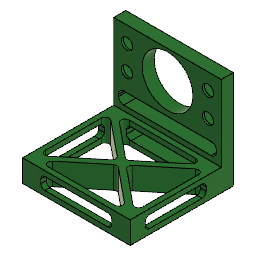
design "LGR Height Extension"
Autodesk Fusion 360 part; units mm, degrees
sketch "Sketch1" plane through (0, 0, 0) normal (0, 0, 1) x (1, 0, 0)
  line L0 (-28.575, 22.5) -> (28.575, 22.5)
  line L1 (28.575, 22.5) -> (28.575, -22.5)
  line L2 (28.575, -22.5) -> (-28.575, -22.5)
  line L3 (-28.575, -22.5) -> (-28.575, 22.5)
  dimension "d1" = 45
  dimension "d2" = 57.15
  dimension "d7" = 28.575
  dimension "d8" = 22.5
  constraint horizontal L0
  constraint vertical L1
  constraint horizontal L2
  constraint vertical L3
  measures "d1" distance of L0 L2
  measures "d2" distance of L1 L3
  measures "d7" distance of origin L1
  measures "d8" distance of origin L0
extrude "Extrude1" add sketch "Sketch1" along normal blind 1 makes body 1
sketch "Sketch3" plane through (0, 0, 1) normal (0, 0, 1) x (-1, 0, 0)
  line L0 (28.575, 22.5) -> (-28.575, 22.5)
  line L1 (-28.575, 22.5) -> (-28.575, -22.5)
  line L2 (-28.575, -22.5) -> (28.575, -22.5)
  line L3 (28.575, -22.5) -> (28.575, 22.5)
  line L4 (28.575, -22.5) -> (-28.575, -22.5)
  line L5 (-28.575, -22.5) -> (-28.575, -23.5)
  line L6 (-28.575, -23.5) -> (28.575, -23.5)
  line L7 (28.575, -23.5) -> (28.575, -22.5)
  dimension "d9" = 1
  dimension "d10" = 57.15
  constraint horizontal L4
  constraint vertical L5
  constraint horizontal L6
  constraint vertical L7
  constraint coincident L2.end L3.start
  measures "d9" distance of L4 L6
  measures "d10" distance of L5 L7
extrude "Extrude2" add sketch "Sketch3" along normal blind 45 separate body contours L2 L4 L5 L6 L7 makes body 2
extrude "Extrude3" add 1 faces at (-9.525, 23.1667, 1) along direction (0, 0, -1) blind 1 on bodies 2 bodies 1 2
extrude "Extrude4" add 1 faces at (9.525, 23.5, 30.6667) along direction (0, 1, 0) blind 5 on bodies 1 bodies 1
extrude "Extrude5" add 1 faces at (-9.525, 11.5, 0) along direction (0, 0, -1) blind 5 on bodies 1 bodies 1
sketch "Sketch5" plane through (0, 28.5, 0) normal (0, 1, 0) x (-1, 0, 0)
  line L0 (28.575, -5) -> (28.575, 46)
  line L1 (28.575, 46) -> (-28.575, 46)
  line L2 (-28.575, 46) -> (-28.575, -5)
  line L3 (-28.575, -5) -> (28.575, -5)
  point P0 (-20, 30.5)
  point P1 (20, 30.5)
  point P2 (-20, 18.5)
  point P3 (20, 18.5)
  dimension "d28" = 40
  dimension "d29" = 12
  dimension "d31" = 8.575
  dimension "d38" = 23.5
  constraint horizontal P0 P1
  constraint vertical P1 P3
  constraint horizontal P2 P3
  constraint vertical P0 P2
  measures "d28" distance of P0 P1
  measures "d29" distance of P1 P3
  measures "d31" distance of L2 P0
  measures "d38" distance of L3 P2
hole "Hole2" at (20, 28.5, 30.5) at (-20, 28.5, 30.5) at (-20, 28.5, 18.5) at (20, 28.5, 18.5) direction (0, -1, 0) diameter 5.5 depth 6 tip angle 180 counterbore diameter 10 counterbore depth 5 bodies 1
extrude "Extrude6" cut 1 faces at (-28.575, 9.5, -3) along direction (-1, 0, 0) blind 0 and the other way blind 2 on bodies 1 bodies 1
extrude "Extrude7" cut 1 faces at (28.575, 9.5, -3) along direction (1, 0, 0) blind 0 and the other way blind 2 on bodies 1 bodies 1
extrude "Extrude8" cut 1 faces at (-8.8583, 24.5, 46) along direction (0, 0, 1) blind 0 and the other way blind 7.5 on bodies 1 bodies 1
sketch "Sketch6" plane through (0, 28.5, 0) normal (0, 1, 0) x (-1, 0, 0)
  line L0 (26.575, 38.5) -> (-26.575, 38.5)
  line L1 (-26.575, 38.5) -> (-26.575, -5)
  line L2 (-26.575, -5) -> (26.575, -5)
  line L3 (26.575, -5) -> (26.575, 38.5)
  circle A0 centre (20, 18.5) radius 5
  circle A1 centre (-20, 30.5) radius 5
  circle A2 centre (20, 30.5) radius 5
  circle A3 centre (-20, 18.5) radius 5
  circle A4 centre (0, 24.5) radius 12.5
  dimension "d51" = 25
  dimension "d52" = 20
  dimension "d53" = 6
  measures "d51" diameter of A4
  measures "d52" horizontal distance of A3.centre A4.centre
  measures "d53" vertical distance of A2.centre A4.centre
extrude "Extrude9" cut sketch "Sketch6" along normal blind 0 and the other way blind 6 contours A4 bodies 1
sketch "Sketch9" plane through (0, 0, 1) normal (0, 0, 1) x (-1, 0, 0)
  line L0 (-26.575, 22.5) -> (-26.575, -22.5)
  line L1 (-26.575, -22.5) -> (26.575, -22.5)
  line L2 (26.575, -22.5) -> (26.575, 22.5)
  line L3 (26.575, 22.5) -> (-26.575, 22.5)
  line L4 (16.3972, -20) -> (-16.3972, -20)
  line L5 (24.075, -13.7886) -> (24.075, 13.7886)
  line L6 (16.3972, 20) -> (-16.3972, 20)
  line L7 (-24.075, 13.7886) -> (-24.075, -13.7886)
  line L8 (-1.2665, -3.0362) -> (-17.6637, -16.4521)
  line L9 (1.2665, -3.0362) -> (17.6637, -16.4521)
  line L10 (20.8111, -15.3386) -> (3.9009, -1.55)
  line L11 (3.9009, 1.55) -> (20.8111, 15.3386)
  line L12 (17.6637, 16.4521) -> (1.2665, 3.0362)
  line L13 (-1.2665, 3.0362) -> (-17.6637, 16.4521)
  line L14 (-20.8111, 15.3386) -> (-3.9009, 1.55)
  line L15 (-3.9009, -1.55) -> (-20.8111, -15.3386)
  arc A0 (20.8111, -15.3386) -> (24.075, -13.7886) centre (22.075, -13.7886) ccw
  arc A1 (3.9009, 1.55) -> (3.9009, -1.55) centre (5.1648, 0) ccw
  arc A2 (24.075, 13.7886) -> (20.8111, 15.3386) centre (22.075, 13.7886) ccw
  arc A3 (17.6637, 16.4521) -> (16.3972, 20) centre (16.3972, 18) ccw
  arc A4 (-16.3972, 20) -> (-17.6637, 16.4521) centre (-16.3972, 18) ccw
  arc A5 (-1.2665, 3.0362) -> (1.2665, 3.0362) centre (0, 4.5841) ccw
  arc A6 (-3.9009, -1.55) -> (-3.9009, 1.55) centre (-5.1648, 0) ccw
  arc A7 (-20.8111, 15.3386) -> (-24.075, 13.7886) centre (-22.075, 13.7886) ccw
  arc A8 (-24.075, -13.7886) -> (-20.8111, -15.3386) centre (-22.075, -13.7886) ccw
  arc A9 (-17.6637, -16.4521) -> (-16.3972, -20) centre (-16.3972, -18) ccw
  arc A10 (16.3972, -20) -> (17.6637, -16.4521) centre (16.3972, -18) ccw
  arc A11 (1.2665, -3.0362) -> (-1.2665, -3.0362) centre (0, -4.5841) ccw
  point P0 (22, -20)
  point P1 (-22, -20)
  point P2 (24.075, -18)
  point P3 (24.075, 18)
  point P4 (22, 20)
  point P5 (-22, 20)
  point P6 (-24.075, 18)
  point P7 (-24.075, -18)
  point P8 (0, -2)
  point P9 (-2, 0)
  point P10 (0, 2)
  point P11 (2, 0)
  dimension "d93" = 44
  dimension "d94" = 44
  dimension "d95" = 36
  dimension "d96" = 36
  dimension "d97" = 22
  dimension "d98" = 22
  dimension "d99" = 18
  dimension "d100" = 18
  dimension "d101" = 2.5
  dimension "d102" = 2.5
  dimension "d103" = 2.5
  dimension "d104" = 2.5
  dimension "d105" = 2
  dimension "d112" = 2
  constraint horizontal L4
  constraint parallel L2 L5
  constraint horizontal L6
  constraint parallel L0 L7
  constraint coincident P2 L10
  constraint coincident P2 L5
  constraint tangent L10 A0
  constraint tangent L5 A0
  constraint tangent L10 A1
  constraint tangent L11 A1
  constraint equal A0 A1
  constraint coincident P3 L11
  constraint coincident P3 L5
  constraint tangent L11 A2
  constraint tangent L5 A2
  constraint equal A0 A2
  constraint coincident P4 L12
  constraint coincident P4 L6
  constraint tangent L12 A3
  constraint tangent L6 A3
  constraint equal A0 A3
  constraint coincident P5 L6
  constraint coincident P5 L13
  constraint tangent L6 A4
  constraint tangent L13 A4
  constraint equal A0 A4
  constraint tangent L13 A5
  constraint tangent L12 A5
  constraint equal A0 A5
  constraint tangent L14 A6
  constraint tangent L15 A6
  constraint equal A0 A6
  constraint coincident P6 L14
  constraint coincident P6 L7
  constraint tangent L14 A7
  constraint tangent L7 A7
  constraint equal A0 A7
  constraint coincident P7 L7
  constraint coincident P7 L15
  constraint tangent L7 A8
  constraint tangent L15 A8
  constraint equal A0 A8
  constraint coincident P1 L8
  constraint coincident P1 L4
  constraint tangent L8 A9
  constraint tangent L4 A9
  constraint equal A0 A9
  constraint coincident P0 L9
  constraint coincident P0 L4
  constraint tangent L9 A10
  constraint tangent L4 A10
  constraint equal A0 A10
  constraint tangent L9 A11
  constraint tangent L8 A11
  measures "d93" distance of P0 P1
  measures "d94" distance of P4 P5
  measures "d95" distance of P6 P7
  measures "d96" distance of P2 P3
  measures "d97" horizontal distance of origin P1
  measures "d98" horizontal distance of origin P4
  measures "d99" vertical distance of origin P6
  measures "d100" vertical distance of origin P2
  measures "d101" distance of L3 L6
  measures "d102" distance of L0 L7
  measures "d103" distance of L2 L5
  measures "d104" distance of L1 L4
  measures "d105" radius of A0
  measures "d112" radius of A11
extrude "Extrude11" cut sketch "Sketch9" along normal blind 0 and the other way blind 6 contours L4 L8 L9 A9 A10 A11 | L5 L10 L11 A0 A1 A2 | L6 L12 L13 A3 A4 A5 | L7 L14 L15 A6 A7 A8 bodies 1
sketch "Sketch10" plane through (0, 22.5, 0) normal (0, -1, 0) x (1, 0, 0)
  circle A0 centre (0, 24.5) radius 12.5
  line L0 (26.575, 38.5) -> (-26.575, 38.5)
  line L1 (-26.575, 38.5) -> (-26.575, 1)
  line L2 (-26.575, 1) -> (26.575, 1)
  line L3 (26.575, 1) -> (26.575, 38.5)
  circle A1 centre (20, 18.5) radius 2.75
  circle A2 centre (-20, 30.5) radius 2.75
  circle A3 centre (20, 30.5) radius 2.75
  circle A4 centre (-20, 18.5) radius 2.75
  line L4 (-21.575, 9.5) -> (21.575, 9.5)
  line L5 (24.075, 7) -> (24.075, 6)
  line L6 (21.575, 3.5) -> (-21.575, 3.5)
  line L7 (-24.075, 6) -> (-24.075, 7)
  arc A5 (-21.575, 9.5) -> (-24.075, 7) centre (-21.575, 7) ccw
  arc A6 (-24.075, 6) -> (-21.575, 3.5) centre (-21.575, 6) ccw
  arc A7 (21.575, 3.5) -> (24.075, 6) centre (21.575, 6) ccw
  arc A8 (24.075, 7) -> (21.575, 9.5) centre (21.575, 7) ccw
  dimension "d113" = 2.5
  dimension "d114" = 2.5
  dimension "d115" = 2.5
  dimension "d116" = 15
  dimension "d117" = 2.5
  constraint horizontal L4
  constraint vertical L5
  constraint horizontal L6
  constraint vertical L7
  constraint tangent L4 A5
  constraint tangent L7 A5
  constraint tangent L7 A6
  constraint tangent L6 A6
  constraint equal A5 A6
  constraint tangent L6 A7
  constraint tangent L5 A7
  constraint equal A5 A7
  constraint tangent L5 A8
  constraint tangent L4 A8
  constraint equal A5 A8
  measures "d113" distance of L2 L6
  measures "d114" distance of L1 L7
  measures "d115" distance of L3 L5
  measures "d116" distance of A0.centre L4
  measures "d117" radius of A5
extrude "Extrude13" cut sketch "Sketch10" against normal blind 6 contours L4 L5 L6 L7 A5 A6 A7 A8 bodies 1
extrude "Extrude14" add 1 faces at (5.4657, 25.6667, -5) along direction (0, 0, -1) blind 5 on bodies 1 bodies 1
sketch "Sketch13" plane through (26.575, 0, 0) normal (1, 0, 0) x (0, 1, 0)
  line L0 (28.5, 38.5) -> (22.5, 38.5)
  line L1 (22.5, 38.5) -> (22.5, 1)
  line L2 (22.5, 1) -> (-22.5, 1)
  line L3 (-22.5, 1) -> (-22.5, -10)
  line L4 (-22.5, -10) -> (28.5, -10)
  line L5 (28.5, -10) -> (28.5, 38.5)
  line L6 (-13, -1.5) -> (13, -1.5)
  line L7 (15, -3.5) -> (15, -5.5)
  line L8 (13, -7.5) -> (-13, -7.5)
  line L9 (-15, -5.5) -> (-15, -3.5)
  arc A0 (-13, -1.5) -> (-15, -3.5) centre (-13, -3.5) ccw
  arc A1 (-15, -5.5) -> (-13, -7.5) centre (-13, -5.5) ccw
  arc A2 (13, -7.5) -> (15, -5.5) centre (13, -5.5) ccw
  arc A3 (15, -3.5) -> (13, -1.5) centre (13, -3.5) ccw
  dimension "d124" = 2.5
  dimension "d125" = 2.5
  dimension "d126" = 7.5
  dimension "d127" = 13.5
  dimension "d128" = 2
  constraint horizontal L6
  constraint vertical L7
  constraint horizontal L8
  constraint vertical L9
  constraint tangent L6 A0
  constraint tangent L9 A0
  constraint tangent L9 A1
  constraint tangent L8 A1
  constraint equal A0 A1
  constraint tangent L8 A2
  constraint tangent L7 A2
  constraint equal A0 A2
  constraint tangent L7 A3
  constraint tangent L6 A3
  constraint equal A0 A3
  measures "d124" distance of L2 L6
  measures "d125" distance of L4 L8
  measures "d126" distance of L3 L9
  measures "d127" distance of L5 L7
  measures "d128" radius of A0
extrude "Extrude15" cut sketch "Sketch13" against normal blind 4 contours L6 L7 L8 L9 A0 A1 A2 A3 bodies 1